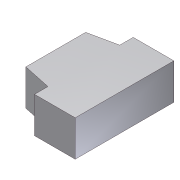
# Autodesk Inventor part: LED_LTST-S270KFKT
Saved by Autodesk Inventor 2014 SP1 (Build 180222100, 222)
## iProperties
Created: 2013-08-12
Part Number: LED_LTST-S270KFKT
Document SubType Name: Modeling
Designer: Robert Davis
Density: 1 g/cm^3
Material: Generic
Appearance: Default
Author: Robert Davis
Autodesk Inventor part; units mm, degrees
ref_plane "YZ Plane" through (0, 0, 0) normal (1, 0, 0) x (0, 1, 0)
ref_plane "XZ Plane" through (0, 0, 0) normal (0, 1, 0) x (-1, 0, 0)
ref_plane "XY Plane" through (0, 0, 0) normal (0, 0, 1) x (1, 0, 0)
sketch "Sketch1" plane through (0, 0, 0) normal (0, 0, 1) x (1, 0, 0)
  line L0 (0, 0) -> (21.5711, 0)
  line L1 (-0.68, 0.825) -> (0, 0.825)
  line L2 (0, 0.825) -> (0, -0.825)
  line L3 (0, -0.825) -> (-0.68, -0.825)
  line L4 (-0.68, 0.6) -> (-1.15, 0.5)
  line L5 (-1.15, 0.5) -> (-1.15, -0.5)
  line L6 (-1.15, -0.5) -> (-0.68, -0.6)
  line L7 (-0.68, -0.825) -> (-0.68, -0.6)
  line L8 (-0.68, 0.6) -> (-0.68, 0.825)
  point P0 (0, 0)
  dimension "d2" = 0.68
  dimension "d3" = 1.65
  dimension "d4" = 1.2
  dimension "d5" = 1
  dimension "d6" = 1.15
  constraints: 18 end point, 4 vertical, 2 horizontal, 1 coincident, 1 midpoint, 2 other
  measures "d2" distance of L1.start L1.end
  measures "d3" distance of L1.end L2.end
  measures "d4" distance of L6.end L4.start
  measures "d5" distance of L4.end L5.end
  measures "d6" distance between parallel lines of L2 L5
extrude "Extrusion1" add sketch "Sketch1" along normal mid plane 0.6
body "Solid1"
